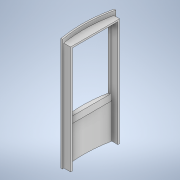
# Autodesk Inventor part: facet
Saved by Autodesk Inventor 2022 (Build 260153000, 153)
## iProperties
Created: 2023-03-27
Part Number: facet
Material: Generic
Document SubType Name: Modeling
Designer: emp
Density: 1 g/cm^3
Appearance: Default
Author: emp
Autodesk Inventor part; units mm, degrees
ref_plane "YZ Plane" through (0, 0, 0) normal (1, 0, 0) x (0, 1, 0)
ref_plane "XZ Plane" through (0, 0, 0) normal (0, 1, 0) x (-1, 0, 0)
ref_plane "XY Plane" through (0, 0, 0) normal (0, 0, 1) x (1, 0, 0)
sketch "Sketch1" plane through (0, 0, 0) normal (0, 1, 0) x (-1, 0, 0)
  line L0 (0, -37.5) -> (4.5, -37.5) construction
  line L1 (0, 0) -> (2, 0) construction
  line L2 (4.5, -37.5) -> (6.5, -37.5) construction
  line L3 (0, -75) -> (2, -75) construction
  arc A0 (2.4733, -73) -> (3.9166, -9) centre (-152, -37.5) ccw
  line L4 (1.9166, -9) -> (3.9166, -9)
  line L5 (0, -73) -> (2.4733, -73)
  line L6 (0, -15) -> (2.8949, -15) construction
  line L7 (0, -67) -> (1.7305, -67) construction
  line L8 (0, -69) -> (1.3383, -69) construction
  line L9 (1.3383, -69) -> (1.3383, -67)
  line L10 (1.3383, -67) -> (1.7305, -67)
  arc A1 (2.2393, -10.8253) -> (1.9166, -9) centre (-154, -37.5) ccw
  arc A2 (0.4733, -73) -> (0.9193, -71) centre (-154, -37.5) ccw
  arc A3 (1.7305, -67) -> (2.8949, -15) centre (-154, -37.5) ccw
  line L11 (-6.1617, -13) -> (-6.1617, -11)
  line L12 (-6.1617, -11) -> (-6.1617, -10.8253)
  line L13 (-6.1617, -10.8253) -> (2.2393, -10.8253)
  line L14 (1.3383, -67) -> (1.3383, -5.3327) construction
  line L15 (2.8949, -15) -> (1.3383, -15) construction
  line L16 (2.8949, -15) -> (1.3383, -15)
  line L17 (1.3383, -15) -> (1.3383, -13)
  line L18 (1.3383, -13) -> (-6.1617, -13)
  line L19 (1.3383, -69) -> (-6.1617, -69)
  line L20 (-6.1617, -69) -> (-6.1617, -71)
  line L21 (-6.1617, -71) -> (0.9193, -71)
  arc A4 (2.8949, -15) -> (2.2393, -10.8253) centre (-154, -37.5) ccw
  line L22 (1.3383, -13) -> (2.595, -13)
  arc A5 (0.9193, -71) -> (1.7305, -67) centre (-154, -37.5) ccw
  line L23 (1.3383, -15) -> (1.3383, -67)
  line L24 (-6.1617, -13) -> (-6.1617, -69)
  line L25 (2.8949, -15) -> (4.8949, -15)
  line L26 (1.7305, -67) -> (3.7305, -67)
  point P0 (0, -7)
  point P1 (2, 0)
  point P2 (0, -9)
  point P3 (0, -41)
  point P4 (0, -13)
  dimension "d14" = 75
  dimension "d15" = 4.5
  dimension "d16" = 68
  dimension "d17" = 2
  dimension "d18" = 2
  dimension "d19" = 2
  dimension "d20" = 2
  dimension "d21" = 2
  dimension "d22" = 32
  dimension "d23" = 26
  dimension "d24" = 26
  dimension "d26" = 28
  dimension "d27" = 28
  dimension "d29" = 2
  dimension "d30" = 7.5
  dimension "d31" = 7.5
  dimension "d32" = 2
  constraints: 54 end point, 17 point on circle, 10 horizontal, 6 centre point, 6 point on line, 5 coincident, 5 perpendicular, 4 collinear, 3 parallel, 1 concentric, 1 vertical
  measures "d14" distance of L1.start L3.start
  measures "d15" distance of L0.start L0.end
  measures "d16" distance of L3.start point (0, -7)
  measures "d17" distance of L1.start L1.end
  measures "d18" distance of L0.end L2.end
  measures "d19" distance of L3.start L3.end
  measures "d20" distance of point (0, -75) L5.start
  measures "d21" distance of point (0, -9) point (0, -7)
  measures "d22" distance of L5.start point (0, -41)
  measures "d23" distance of L7.start point (0, -41)
  measures "d24" distance of point (0, -41) L6.start
  measures "d26" distance of L8.start point (0, -41)
  measures "d27" distance of point (0, -41) point (0, -13)
  measures "d29" distance of L11.start L11.end
  measures "d30" distance of L11.start L17.end
  measures "d31" distance of L8.end L19.end
  measures "d32" distance of L19.end L20.end
extrude "Extrusion1" add sketch "Sketch1" along normal blind 138 contours L5 A2 A5 L26 A0 | L26 A3 L25 A0 | L25 A4 A1 L4 A0
extrude "Extrusion2" add sketch "Sketch1" along normal blind 133 contours A5 L9 L10 | L10 L23 L16 A3 | L21 L20 L19 A5 | L16 L17 L22 A4 | L9 L19 L24 L18 L17 L23 | L22 L18 L11 L12 L13 A4
extrude "Extrusion3" cut sketch "Sketch1" along normal blind 131 contours L10 L23 L16 A3 | L9 L19 L24 L18 L17 L23
extrude "Extrusion4" cut sketch "Sketch1" along normal blind 129 contours L26 A3 L25 A0
extrude "Extrusion5" add sketch "Sketch1" along normal blind 131 contours L10 L23 L16 A3
extrude "Extrusion6" cut sketch "Sketch1" along normal blind 129 contours L10 L23 L16 A3
extrude "Extrusion7" add sketch "Sketch1" along normal blind 51 contours L26 A3 L25 A0
extrude "Extrusion8" add sketch "Sketch1" along normal blind 51 contours L10 L23 L16 A3
extrude "Extrusion9" cut sketch "Sketch1" along normal blind 43 contours A5 L9 L10 | L10 L23 L16 A3 | L16 L17 L22 A4 | L9 L19 L24 L18 L17 L23
body "Solid1"
